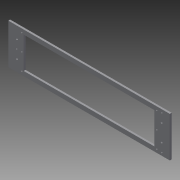
# Autodesk Inventor part: 300 mm core xy gantry
Saved by Autodesk Inventor 2014 SP1 (Build 180222100, 222)
## iProperties
Created: 2014-09-28
Part Number: 300 mm core xy gantry
Material: Generic
Document SubType Name: Modeling
Designer: Mon
Density: 1 g/cm^3
Appearance: Default
Author: Mon
Autodesk Inventor part; units mm, degrees
ref_plane "YZ Plane" through (0, 0, 0) normal (1, 0, 0) x (0, 1, 0)
ref_plane "XZ Plane" through (0, 0, 0) normal (0, 1, 0) x (-1, 0, 0)
ref_plane "XY Plane" through (0, 0, 0) normal (0, 0, 1) x (1, 0, 0)
sketch "Sketch1" plane through (0, 0, 0) normal (0, 1, 0) x (-1, 0, 0)
  line L0 (381.1493, 61.7688) -> (30.4355, 61.7688)
  line L1 (380.945, 412.5458) -> (381.1493, 61.7688)
  line L2 (30.2312, 412.5458) -> (380.945, 412.5458)
  line L3 (30.4355, 61.7688) -> (30.4355, 412.5458)
  arc A0 (0.0979, 16.0688) -> (16.0979, 0.0688) centre (16.0979, 16.0688) ccw
  line L4 (0.1355, 16.0688) -> (-0.0688, 429.5458)
  arc A1 (15.9312, 445.5458) -> (-0.0688, 429.5458) centre (15.9312, 429.5458) ccw
  line L5 (15.9312, 445.5458) -> (395.245, 445.5458)
  arc A2 (411.245, 429.5458) -> (395.245, 445.5458) centre (395.245, 429.5458) ccw
  line L6 (411.245, 429.5458) -> (411.4493, 16.0688)
  arc A3 (395.4117, 0.0688) -> (411.4117, 16.0688) centre (395.4117, 16.0688) ccw
  line L7 (395.4117, 0.0688) -> (16.0979, 0.0688)
  arc A4 (21.3729, 6.5688) -> (25.1229, 6.5688) centre (23.2479, 6.5688) ccw
  line L8 (25.1229, 10.5688) -> (25.1229, 6.5688)
  arc A5 (25.1229, 10.5688) -> (21.3729, 10.5688) centre (23.2479, 10.5688) ccw
  line L9 (21.3729, 6.5688) -> (21.3729, 10.5688)
  arc A6 (52.3729, 6.5688) -> (56.1229, 6.5688) centre (54.2479, 6.5688) ccw
  line L10 (56.1229, 10.5688) -> (56.1229, 6.5688)
  arc A7 (56.1229, 10.5688) -> (52.3729, 10.5688) centre (54.2479, 10.5688) ccw
  line L11 (52.3729, 6.5688) -> (52.3729, 10.5688)
  arc A8 (21.3729, 37.5688) -> (25.1229, 37.5688) centre (23.2479, 37.5688) ccw
  line L12 (25.1229, 41.5688) -> (25.1229, 37.5688)
  arc A9 (25.1229, 41.5688) -> (21.3729, 41.5688) centre (23.2479, 41.5688) ccw
  line L13 (21.3729, 37.5688) -> (21.3729, 41.5688)
  arc A10 (52.3729, 37.5688) -> (56.1229, 37.5688) centre (54.2479, 37.5688) ccw
  line L14 (56.1229, 41.5688) -> (56.1229, 37.5688)
  arc A11 (56.1229, 41.5688) -> (52.3729, 41.5688) centre (54.2479, 41.5688) ccw
  line L15 (52.3729, 37.5688) -> (52.3729, 41.5688)
  arc A12 (26.7479, 22.0688) -> (50.7479, 22.0688) centre (38.7479, 22.0688) ccw
  line L16 (50.7479, 26.0688) -> (50.7479, 22.0688)
  arc A13 (50.7479, 26.0688) -> (26.7479, 26.0688) centre (38.7479, 26.0688) ccw
  line L17 (26.7479, 22.0688) -> (26.7479, 26.0688)
  arc A14 (355.4177, 6.5688) -> (359.1677, 6.5688) centre (357.2927, 6.5688) ccw
  line L18 (359.1677, 10.5688) -> (359.1677, 6.5688)
  arc A15 (359.1677, 10.5688) -> (355.4177, 10.5688) centre (357.2927, 10.5688) ccw
  line L19 (355.3867, 6.5688) -> (355.3867, 10.5688)
  arc A16 (386.3692, 6.5688) -> (390.1192, 6.5688) centre (388.2442, 6.5127) ccw
  arc A17 (386.3762, 37.5688) -> (390.1262, 37.5688) centre (388.2512, 37.5688) ccw
  line L20 (390.1262, 41.5688) -> (390.1262, 37.5688)
  arc A18 (390.1367, 41.5688) -> (386.3867, 41.5688) centre (388.2617, 41.5688) ccw
  line L21 (386.3762, 37.5688) -> (386.3762, 41.5688)
  arc A19 (355.3676, 37.5688) -> (359.1176, 37.5688) centre (357.2426, 37.5688) ccw
  line L22 (359.1176, 41.5688) -> (359.1176, 37.5688)
  arc A20 (359.1367, 41.5688) -> (355.3867, 41.5688) centre (357.2617, 41.5688) ccw
  line L23 (355.3676, 37.5688) -> (355.3676, 41.5688)
  arc A21 (360.7225, 22.0688) -> (384.7225, 22.0688) centre (372.7225, 22.0688) ccw
  line L24 (384.7225, 26.0688) -> (384.7225, 22.0688)
  arc A22 (384.7617, 26.0688) -> (360.7617, 26.0688) centre (372.7617, 26.0688) ccw
  line L25 (360.7225, 22.0688) -> (360.7225, 26.0688)
  circle A23 centre (50.1812, 420.5458) radius 2.1
  circle A24 centre (38.5812, 435.5458) radius 2.1
  circle A25 centre (372.595, 435.5458) radius 2.1
  circle A26 centre (360.995, 420.5458) radius 2.1
  circle A27 centre (25.8187, 418.0458) radius 1.6
  circle A28 centre (66.8187, 418.0458) radius 1.6
  circle A29 centre (205.5881, 418.0458) radius 1.6
  circle A30 centre (344.3575, 418.0458) radius 1.6
  circle A31 centre (385.3575, 418.0458) radius 1.6
  circle A32 centre (385.3575, 56.2688) radius 1
  circle A33 centre (344.3575, 56.2688) radius 1
  circle A34 centre (205.5881, 56.2688) radius 1
  circle A35 centre (66.8187, 56.2688) radius 1
  circle A36 centre (25.8187, 56.2688) radius 1
  arc A37 (390.1367, 10.5688) -> (386.3867, 10.5688) centre (388.2617, 10.5688) ccw
  line L26 (378.8577, 179.5323) -> (32.233, 179.5323)
  circle A38 centre (60.683, 222.8073) radius 1.6
  circle A39 centre (60.683, 258.6198) radius 1.6
  circle A40 centre (60.683, 186.9948) radius 1.6
  circle A41 centre (350.4077, 186.9948) radius 1.6
  circle A42 centre (350.4077, 222.8073) radius 1.6
  circle A43 centre (350.4077, 258.6198) radius 1.6
  circle A44 centre (49.883, 185.8823) radius 1.6
  circle A45 centre (49.883, 259.7323) radius 1.6
  circle A46 centre (361.2077, 222.8073) radius 1.6
  line L27 (378.8577, 266.0823) -> (378.8577, 179.5323)
  line L28 (345.9077, 256.5573) -> (345.9077, 189.0573)
  line L29 (65.183, 256.5573) -> (345.9077, 256.5573)
  line L30 (65.183, 189.0573) -> (65.183, 256.5573)
  line L31 (345.9077, 189.0573) -> (65.183, 189.0573)
  line L32 (32.233, 179.5323) -> (32.233, 266.0823)
  line L33 (32.233, 266.0823) -> (378.8577, 266.0823)
  circle A47 centre (50.183, 204.5073) radius 2.1
  circle A48 centre (360.9077, 204.5073) radius 2.1
  circle A49 centre (360.9077, 241.1073) radius 2.1
  circle A50 centre (50.183, 241.1073) radius 2.1
  line L34 (224.6381, 203.7573) -> (186.5381, 203.7573)
  line L35 (224.6381, 207.8163) -> (224.6381, 203.7573)
  arc A51 (226.0481, 209.3136) -> (224.6381, 207.8163) centre (226.1381, 207.8163) ccw
  arc A52 (226.0481, 209.3136) -> (226.0481, 216.301) centre (225.8381, 212.8073) ccw
  arc A53 (224.6381, 217.7983) -> (226.0481, 216.301) centre (226.1381, 217.7983) ccw
  arc A54 (226.0481, 229.3136) -> (224.6381, 227.8163) centre (226.1381, 227.8163) ccw
  arc A55 (226.0481, 229.3136) -> (226.0481, 236.301) centre (225.8381, 232.8073) ccw
  arc A56 (224.6381, 237.7983) -> (226.0481, 236.301) centre (226.1381, 237.7983) ccw
  line L36 (186.5381, 241.8573) -> (224.6381, 241.8573)
  line L37 (186.5381, 237.7983) -> (186.5381, 241.8573)
  arc A57 (185.1281, 236.301) -> (186.5381, 237.7983) centre (185.0381, 237.7983) ccw
  arc A58 (185.1281, 236.301) -> (185.1281, 229.3136) centre (185.3381, 232.8073) ccw
  arc A59 (186.5381, 227.8163) -> (185.1281, 229.3136) centre (185.0381, 227.8163) ccw
  arc A60 (185.1281, 216.301) -> (186.5381, 217.7983) centre (185.0381, 217.7983) ccw
  arc A61 (185.1281, 216.301) -> (185.1281, 209.3136) centre (185.3381, 212.8073) ccw
  arc A62 (186.5381, 207.8163) -> (185.1281, 209.3136) centre (185.0381, 207.8163) ccw
  line L38 (173.8381, 254.5573) -> (237.3381, 254.5573)
  line L39 (237.3381, 254.5573) -> (237.3381, 191.0573)
  line L40 (237.3381, 191.0573) -> (173.8381, 191.0573)
  line L41 (173.8381, 191.0573) -> (173.8381, 254.5573)
  circle A63 centre (180.1881, 196.9948) radius 0.875
  circle A64 centre (230.9881, 196.9948) radius 0.875
  circle A65 centre (230.9881, 248.6198) radius 0.875
  circle A66 centre (180.1881, 248.6198) radius 0.875
  circle A67 centre (177.8381, 232.8073) radius 0.875
  circle A68 centre (233.3381, 232.8073) radius 0.875
  circle A69 centre (233.3381, 212.8073) radius 0.875
  circle A70 centre (177.8381, 212.8073) radius 0.875
  line L42 (186.5381, 203.7573) -> (186.5381, 207.8163)
  line L43 (186.5381, 217.7983) -> (186.5381, 227.8163)
  line L44 (224.6381, 241.8573) -> (224.6381, 237.7983)
  line L45 (224.6381, 227.8163) -> (224.6381, 217.7983)
  line L46 (390.1367, 10.5688) -> (390.1367, 6.5605)
  line L47 (386.3867, 10.5688) -> (386.3867, 6.2509)
  circle A71 centre (136.8187, 56.2688) radius 1
  circle A72 centre (273.8511, 56.2688) radius 1
  circle A73 centre (274.3575, 418.0458) radius 1.6
  circle A74 centre (136.8187, 418.0458) radius 1.6
  point P0 (0, 0)
  constraints: 96 end point, 75 centre point, 73 point on circle, 1 point on line
extrude "Extrusion1" add sketch "Sketch1" along normal blind 4 contours L26 L32 L33 L27
body "Solid1"
